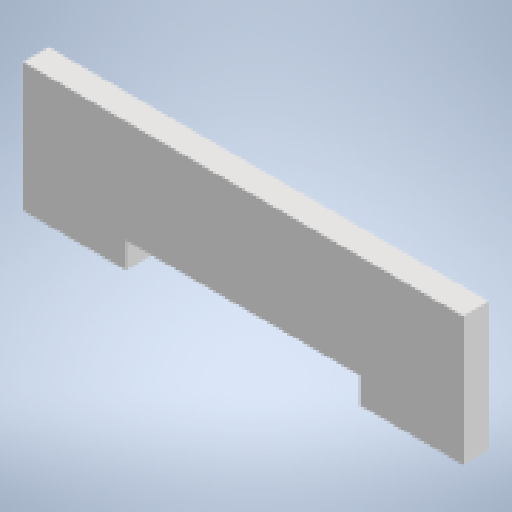
# Autodesk Inventor part: 皿_壁
Saved by Autodesk Inventor 2024.1 (Build 281209000, 209)
## iProperties
Created: 2024-05-01
Part Number: 皿_壁
Material: 一般
Document SubType Name: Modeling
Designer: hibik
Density: 1 g/cm^3
Appearance: 既定
Author: hibik
Autodesk Inventor part; units mm, degrees
ref_plane "YZ Plane" through (0, 0, 0) normal (1, 0, 0) x (0, 1, 0)
ref_plane "XZ Plane" through (0, 0, 0) normal (0, 1, 0) x (-1, 0, 0)
ref_plane "XY Plane" through (0, 0, 0) normal (0, 0, 1) x (1, 0, 0)
sketch "スケッチ1" plane through (0, 0, 0) normal (0, 0, 1) x (1, 0, 0)
  line L0 (0, 0) -> (50, 0)
  line L1 (50, 0) -> (50, 10)
  line L2 (50, 10) -> (0, 10)
  line L3 (0, 10) -> (0, 0)
  dimension "d0" = 50
  dimension "d1" = 10
  constraints: 8 end point, 2 parallel, 1 horizontal, 1 perpendicular
  measures "d0" distance of L2.end L1.end
  measures "d1" distance of L1.end L0.end
extrude "押し出し1" add sketch "スケッチ1" along normal blind 2.5
sketch "スケッチ2" plane through (0, 0, 2.5) normal (0, 0, 1) x (1, 0, 0)
  line L0 (10, -2.5) -> (0, -2.5) projected
  line L1 (10, 0) -> (10, -2.5) projected
  line L2 (0, 0) -> (10, 0) projected
  line L3 (0, 0) -> (0, -2.5) projected
  line L4 (42.7436, -2.5) -> (32.7436, -2.5) projected
  line L5 (42.7436, 0) -> (42.7436, -2.5) projected
  line L6 (32.7436, 0) -> (42.7436, 0) projected
  line L7 (32.7436, 0) -> (32.7436, -2.5) projected
  line L8 (42.7436, 0) -> (42.7436, 10)
  line L9 (50, 0) -> (50, 10) projected
  line L10 (50, 10) -> (0, 10) projected
  line L11 (0, 10) -> (0, 0) projected
  line L12 (0, 0) -> (50, 0) projected
  constraints: 2 end point, 1 vertical
extrude "押し出し2" cut sketch "スケッチ2" against normal through all contours L8 L10 L9 L12
sketch "スケッチ3" plane through (0, 0, 2.5) normal (0, 0, 1) x (1, 0, 0)
  line L0 (10, -2.5) -> (0, -2.5) projected
  line L1 (10, 0) -> (10, -2.5) projected
  line L2 (0, 0) -> (10, 0) projected
  line L3 (0, 0) -> (0, -2.5) projected
  line L4 (42.7436, -2.5) -> (32.7436, -2.5) projected
  line L5 (42.7436, 0) -> (42.7436, -2.5) projected
  line L6 (32.7436, 0) -> (42.7436, 0) projected
  line L7 (32.7436, 0) -> (32.7436, -2.5) projected
extrude "押し出し3" add sketch "スケッチ3" against normal up to surface (2.5 mm away)
